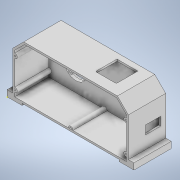
# Autodesk Inventor part: carcaça corpo
Saved by Autodesk Inventor 2022.1 (Build 261234020, 234B)
## iProperties
Created: 2023-09-12
Part Number: carcaça corpo
Material: Generic
Document SubType Name: Modeling
Designer: SENAI
Density: 1 g/cm^3
Appearance: Default
Author: SENAI
Autodesk Inventor part; units mm, degrees
ref_plane "YZ Plane" through (0, 0, 0) normal (1, 0, 0) x (0, 1, 0)
sketch "Sketch1" plane through (0, 0, 0) normal (0, 0, 1) x (1, 0, 0)
  line L0 (0, 0) -> (0, 25)
  line L1 (0, 25) -> (22.3, 25)
  line L2 (0, 0) -> (59, 0)
  line L3 (59, 0) -> (59, 7.5)
  line L4 (59, 7.5) -> (445.6, 7.5)
  line L5 (445.6, 7.5) -> (445.6, 0)
  line L6 (445.6, 0) -> (504.6, 0)
  line L7 (504.6, 0) -> (504.6, 25)
  line L8 (504.6, 25) -> (482.3, 25)
  line L9 (22.3, 25) -> (22.3, 222.5)
  line L10 (482.3, 25) -> (482.3, 222.5)
  line L11 (482.3, 222.5) -> (22.3, 222.5)
  point P0 (22.3, 7.5)
  dimension "d2" = 25
  dimension "d3" = 22.3
  dimension "d4" = 59
  dimension "d5" = 7.5
  dimension "d6" = 386.6
  dimension "d7" = 59
  dimension "d8" = 25
  dimension "d9" = 22.3
  dimension "d10" = 215
  dimension "d11" = 197.5
  dimension "d12" = 482.3
  constraints: 24 end point, 5 perpendicular, 3 vertical, 2 horizontal, 2 point on line, 1 parallel
  measures "d2" distance of L0.start L0.end
  measures "d3" distance of L1.end L0.end
  measures "d4" distance of L0.start L2.end
  measures "d5" distance of L2.end L3.end
  measures "d6" distance of L3.end L4.end
  measures "d7" distance of L5.end L6.end
  measures "d8" distance of L6.end L7.end
  measures "d9" distance of L7.end L8.end
  measures "d10" distance of point (22.3, 7.5) L9.end
  measures "d11" distance between parallel lines of L8 L11
  measures "d12" distance from line of point (22.3, 7.5) L7
extrude "Extrusion1" add sketch "Sketch1" along normal blind 148.5
sketch "Sketch2" plane through (0, 0, 148.5) normal (0, 0, 1) x (1, 0, 0)
  line L0 (482.3, 222.5) -> (22.3, 222.5) projected
  line L1 (59, 7.5) -> (445.6, 7.5) projected
  line L2 (22.3, 222.5) -> (22.3, 25) projected
  line L3 (482.3, 25) -> (482.3, 222.5) projected
  circle A0 centre (252.3, 213.552) radius 3.25
  circle A1 centre (252.3, 16.448) radius 3.25
  arc A2 (243.164, 215) -> (261.436, 215) centre (252.3, 213.552) ccw
  arc A3 (261.436, 15) -> (243.164, 15) centre (252.3, 16.448) ccw
  line L4 (68.9066, 215) -> (243.164, 215)
  line L5 (261.436, 215) -> (435.6934, 215)
  line L6 (474.8, 15) -> (261.436, 15)
  line L7 (243.164, 15) -> (29.8, 15)
  circle A4 centre (31.248, 39.5844) radius 3.25
  arc A5 (29.8, 30.4484) -> (29.8, 48.7203) centre (31.248, 39.5844) ccw
  line L8 (29.8, 15) -> (29.8, 30.4484)
  circle A6 centre (473.352, 39.5844) radius 3.25
  arc A7 (474.8, 48.7203) -> (474.8, 30.4484) centre (473.352, 39.5844) ccw
  line L9 (474.8, 30.4484) -> (474.8, 15)
  circle A8 centre (31.248, 156.5844) radius 3.25
  circle A9 centre (473.352, 156.5844) radius 3.25
  arc A10 (29.8, 147.4484) -> (29.8, 165.7203) centre (31.248, 156.5844) ccw
  arc A11 (474.8, 165.7203) -> (474.8, 147.4484) centre (473.352, 156.5844) ccw
  line L10 (474.8, 175.8934) -> (474.8, 165.7203)
  line L11 (474.8, 147.4484) -> (474.8, 48.7203)
  line L12 (29.8, 48.7203) -> (29.8, 147.4484)
  line L13 (29.8, 165.7203) -> (29.8, 175.8934)
  line L14 (22.3, 222.5) -> (22.3, 179)
  line L15 (22.3, 222.5) -> (65.8, 222.5)
  line L16 (65.8, 222.5) -> (22.3, 179)
  line L17 (29.8, 175.8934) -> (68.9066, 215)
  line L18 (482.3, 222.5) -> (482.3, 179)
  line L19 (482.3, 222.5) -> (438.8, 222.5)
  line L20 (438.8, 222.5) -> (482.3, 179)
  line L21 (474.8, 175.8934) -> (435.6934, 215)
  point P0 (0, 0)
  point P1 (252.3, 123.75)
  point P2 (252.3, 7.5)
  point P3 (252.3, 222.5)
  dimension "d19" = 6.5
  dimension "d20" = 6.5
  dimension "d24" = 6
  dimension "d25" = 6
  dimension "d27" = 7.5
  dimension "d28" = 7.5
  dimension "d29" = 7.5
  dimension "d30" = 7.5
  dimension "d33" = 6.5
  dimension "d36" = 8.948
  dimension "d37" = 8.948
  dimension "d39" = 6.5
  dimension "d42" = 6.5
  dimension "d43" = 6.5
  dimension "d44" = 117
  dimension "d45" = 117
  dimension "d46" = 6
  dimension "d47" = 6
  dimension "d51" = 43.5
  dimension "d52" = 43.5
  dimension "d53" = 7.5
  dimension "d54" = 43.5
  dimension "d55" = 43.5
  dimension "d56" = 7.5
  dimension "d57" = 7.5
  dimension "d58" = 7.5
  dimension "d59" = 7.5
  dimension "d60" = 8.948
  dimension "d61" = 7.5
  dimension "d62" = 7.5
  dimension "d63" = 7.5
  dimension "d64" = 56.7797
  dimension "d65" = 75.0516
  dimension "d66" = 220.864
  dimension "d67" = 220.864
  dimension "d68" = 98.75
  dimension "d69" = 230
  dimension "d70" = 65.9156
  dimension "d71" = 451.052
  dimension "d72" = 182.9156
  constraints: 36 end point, 13 parallel, 12 centre point, 12 point on circle, 6 coincident, 6 perpendicular, 4 point on line, 2 equal radius, 2 horizontal, 2 midpoint
  measures "d19" diameter of A0
  measures "d20" diameter of A1
  measures "d24" radial gap between concentric circles of A2 A0
  measures "d25" radial gap between concentric circles of A3 A1
  measures "d27" distance between parallel lines of L1 L7
  measures "d28" distance between parallel lines of L1 L6
  measures "d29" distance between parallel lines of L0 L4
  measures "d30" distance between parallel lines of L0 L5
  measures "d33" diameter of A4
  measures "d36" distance of point (252.3, 7.5) A1.centre
  measures "d37" distance of point (252.3, 222.5) A2.centre
  measures "d39" diameter of A6
  measures "d42" diameter of A8
  measures "d43" diameter of A9
  measures "d44" distance of A6.centre A9.centre
  measures "d45" distance of A4.centre A8.centre
  measures "d46" radial gap between concentric circles of A10 A8
  measures "d47" radial gap between concentric circles of A11 A9
  measures "d51" distance of L0.end L14.end
  measures "d52" distance of L0.end L15.end
  measures "d53" distance between parallel lines of L17 L16
  measures "d54" distance of L0.start L18.end
  measures "d55" distance of L0.start L19.end
  measures "d56" distance between parallel lines of L20 L21
  measures "d57" distance between parallel lines of L3 L10
  measures "d58" distance between parallel lines of L3 L11
  measures "d59" distance between parallel lines of L3 L9
  measures "d60" distance from line of L3 A6.centre
  measures "d61" distance between parallel lines of L12 L2
  measures "d62" distance between parallel lines of L13 L2
  measures "d63" distance between parallel lines of L8 L2
  measures "d64" distance from line of L10.end L0
  measures "d65" distance from line of L11.start L0
  measures "d66" distance from line of L5.start L3
  measures "d67" distance from line of L6.end L3
  measures "d68" distance from line of point (252.3, 123.75) L0
  measures "d69" distance from line of point (252.3, 123.75) L3
  measures "d70" distance from line of A10.centre L0
  measures "d71" distance from line of A10.centre L3
  measures "d72" distance from line of A5.centre L0
chamfer "Chamfer1" distance 43.5 angle 45 2 edges at (482.3, 222.5, 74.25) (22.3, 222.5, 74.25)
extrude "Extrusion2" cut sketch "Sketch2" against normal blind 136 contours A2 L5 L21 L10 A11 L11 A7 L9 L6 A3 L7 L8 A5 L12 A10 L13 L17 L4
sketch "Sketch6" plane through (0, 0, 0) normal (0, 0, -1) x (-1, 0, 0)
  circle A0 centre (-367.55, 102) radius 45.25
  circle A1 centre (-137.05, 102) radius 45.25
  line L0 (-482.3, 25) -> (-482.3, 179) projected
  circle A2 centre (-367.55, 102) radius 74.5
  circle A3 centre (-137.05, 102) radius 74.5
  point P0 (0, 0)
  point P1 (-251.8, 102)
  dimension "d75" = 90.5
  dimension "d76" = 90.5
  dimension "d84" = 149
  dimension "d85" = 149
  constraints: 4 centre point, 2 coincident
  measures "d75" diameter of A0
  measures "d76" diameter of A1
  measures "d84" diameter of A2
  measures "d85" diameter of A3
extrude "Extrusion3" add sketch "Sketch6" along normal blind 6
fillet "Fillet1" radius 6 2 edges at (442.05, 102, -6) (211.55, 102, -6) inverted yes
sketch "Sketch7" plane through (367.55, 102, 0) normal (0, 0, -1) x (-1, 0, 0)
  circle A0 centre (0, 0) radius 45.25
  circle A1 centre (230.107, 0) radius 45.25
  point P0 (367.55, -102)
  dimension "d89" = 90.5
  constraints: 2 centre point
  measures "d89" diameter of A1
extrude "Extrusion4" cut sketch "Sketch7" against normal through all
sketch "Sketch8" plane through (65.8, 222.5, 0) normal (0, 1, 0) x (1, 0, 0)
  line L0 (227.25, 0) -> (376.25, 0) projected
  line L1 (327.9158, -22) -> (244.9158, -22)
  line L2 (244.9158, -22) -> (244.9158, -108)
  line L3 (244.9158, -108) -> (327.9158, -108)
  line L4 (327.9158, -108) -> (327.9158, -22)
  point P0 (-65.8, 0)
  dimension "d96" = 83
  dimension "d97" = 86
  constraints: 8 end point, 2 perpendicular, 1 horizontal, 1 vertical
  measures "d96" distance of L1.start L1.end
  measures "d97" distance of L1.end L2.end
extrude "Extrusion5" cut sketch "Sketch8" against normal blind 25
fillet "Fillet2" radius 6 2 edges at (393.7158, 218.75, 108) (310.7158, 218.75, 108)
sketch "Sketch9" plane through (0, 0, 148.5) normal (0, 0, 1) x (1, 0, 0)
  point P0 (0, 0)
sketch "Sketch10" plane through (482.3, 25, 148.5) normal (1, 0, 0) x (0, 0, -1)
  line L0 (148.5, 0) -> (0, 0) projected
  line L1 (128.5, 85.323) -> (68, 85.323)
  line L2 (68, 85.323) -> (68, 51)
  line L3 (68, 51) -> (128.5, 51)
  line L4 (128.5, 85.323) -> (128.5, 51)
  point P0 (148.5, -25)
  dimension "d105" = 60.5
  constraints: 8 end point, 2 perpendicular, 1 horizontal
  measures "d105" distance of L1.start L1.end
extrude "Extrusion6" cut sketch "Sketch10" against normal blind 25
ref_plane "Work Plane1" through (348.5647, 215, 148.5) normal (0, 0, 1) x (1, 0, 0)
sketch "Sketch11" plane through (348.5647, 215, 148.5) normal (0, 0, 1) x (1, 0, 0)
  circle A0 centre (-96.2647, -1.448) radius 3.25
  line L0 (90.2353, 7.5) -> (-282.7647, 7.5) projected
  arc A1 (-105.4006, 0) -> (-87.1287, 0) centre (-96.2647, -1.448) ccw projected
  line L1 (-326.2647, -36) -> (-326.2647, -190) projected
  circle A2 centre (-317.3167, -58.4156) radius 3.25
  arc A3 (-318.7647, -67.5516) -> (-318.7647, -49.2797) centre (-317.3167, -58.4156) ccw projected
  circle A4 centre (-317.3167, -175.4156) radius 3.25
  arc A5 (-318.7647, -184.5516) -> (-318.7647, -166.2797) centre (-317.3167, -175.4156) ccw projected
  circle A6 centre (124.7873, -175.4156) radius 3.25
  line L2 (133.7353, -190) -> (133.7353, -36) projected
  arc A7 (126.2353, -166.2797) -> (126.2353, -184.5516) centre (124.7873, -175.4156) ccw projected
  circle A8 centre (124.7873, -58.4156) radius 3.25
  circle A9 centre (-96.2647, -198.552) radius 3.25
  line L3 (-289.5647, -207.5) -> (97.0353, -207.5) projected
  arc A10 (-87.1287, -200) -> (-105.4006, -200) centre (-96.2647, -198.552) ccw projected
  point P0 (-348.5647, -215)
  dimension "d108" = 6.5
  dimension "d109" = 8.948
  dimension "d110" = 6
  dimension "d113" = 6.5
  dimension "d114" = 8.948
  dimension "d116" = 6
  dimension "d117" = 6.5
  dimension "d118" = 8.948
  dimension "d119" = 6
  dimension "d120" = 6.5
  dimension "d121" = 8.948
  dimension "d122" = 6
  dimension "d123" = 6.5
  dimension "d124" = 8.948
  dimension "d125" = 6.5
  dimension "d126" = 8.948
  dimension "d127" = 6
  constraints: 6 centre point
  measures "d108" diameter of A0
  measures "d109" distance from line of L0 A0.centre
  measures "d110" radial gap between concentric circles of A1 A0
  measures "d113" diameter of A2
  measures "d114" distance from line of L1 A2.centre
  measures "d116" radial gap between concentric circles of A3 A2
  measures "d117" diameter of A4
  measures "d118" distance from line of L1 A4.centre
  measures "d119" radial gap between concentric circles of A5 A4
  measures "d120" diameter of A6
  measures "d121" distance from line of L2 A6.centre
  measures "d122" radial gap between concentric circles of A7 A6
  measures "d123" diameter of A8
  measures "d124" distance from line of L2 A8.centre
  measures "d125" diameter of A9
  measures "d126" distance from line of L3 A9.centre
  measures "d127" radial gap between concentric circles of A10 A9
extrude "Extrusion7" cut sketch "Sketch11" against normal blind 10
ref_plane "Work Plane2" through (0, 0, -6.25) normal (0, 0, 1) x (1, 0, 0)
body "Solid1"
